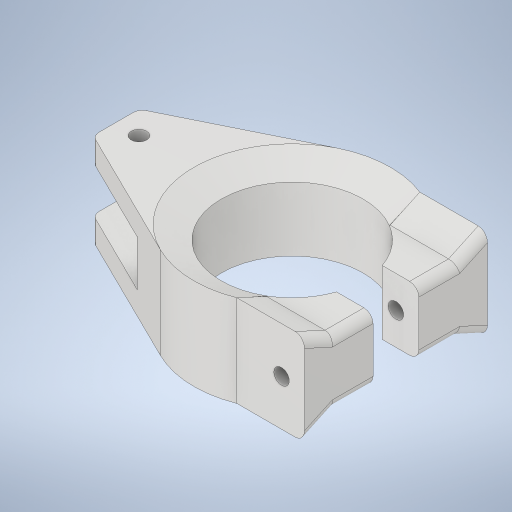
# Autodesk Inventor part: petbottlesfixingparts_sa
Saved by Autodesk Inventor 2024.1 (Build 281209000, 209)
## iProperties
Created: 2019-03-19
Part Number: petbottlesfixingparts_sa
Material: ABS プラスチック
Document SubType Name: Modeling
Designer: shun
Density: 1.06 g/cm^3
Appearance: 滑らか - 白
Author: shun
Autodesk Inventor part; units mm, degrees
ref_plane "YZ Plane" through (0, 0, 0) normal (1, 0, 0) x (0, 1, 0)
ref_plane "XZ Plane" through (0, 0, 0) normal (0, 1, 0) x (-1, 0, 0)
ref_plane "XY Plane" through (0, 0, 0) normal (0, 0, 1) x (1, 0, 0)
sketch "スケッチ1" plane through (0, 0, 0) normal (0, 1, 0) x (-1, 0, 0)
  circle A0 centre (0, 0) radius 15.5 construction
  circle A1 centre (0, 0) radius 21.5 construction
  line L0 (-22.6714, 5) -> (-14.6714, 5)
  line L1 (-14.6714, 5) -> (-14.6714, -5) construction
  line L2 (-14.6714, -5) -> (-22.6714, -5)
  line L3 (-22.6714, -5) -> (-22.6714, 5) construction
  line L4 (-22.6714, 5) -> (-14.6714, -5) construction
  line L5 (-14.6714, 5) -> (-22.6714, -5) construction
  line L6 (0, 0) -> (-18.6714, 0) construction
  line L7 (-22.6714, 5) -> (-22.6714, 20)
  line L8 (-22.6714, 20) -> (-7.8899, 20)
  line L9 (-22.6714, -5) -> (-22.6714, -20)
  line L10 (-22.6714, -20) -> (-7.8899, -20)
  arc A2 (-14.6714, -5) -> (-14.6714, 5) centre (0, 0) ccw
  line L11 (21.5, 0) -> (33.5, 0) construction
  line L12 (0, 0) -> (21.5, 0) construction
  line L13 (33.5, 0) -> (38.5, 0) construction
  line L14 (38.5, 0) -> (38.5, 5)
  line L15 (38.5, 0) -> (38.5, -5)
  line L16 (38.5, 5) -> (9.5018, 19.2864)
  line L17 (38.5, -5) -> (9.5018, -19.2864)
  arc A3 (9.5018, 19.2864) -> (-7.8899, 20) centre (0, 0) ccw
  arc A4 (-7.8899, -20) -> (9.5018, -19.2864) centre (0, 0) ccw
  dimension "d0" = 31
  dimension "d1" = 43
  dimension "d2" = 10
  dimension "d3" = 8
  dimension "d4" = 15
  dimension "d5" = 15
  dimension "d6" = 12
  dimension "d7" = 5
  dimension "d8" = 5
  dimension "d9" = 5
  constraints: 36 end point, 11 point on circle, 6 coincident, 5 horizontal, 4 centre point, 4 perpendicular, 2 midpoint, 2 parallel, 2 tangent, 2 vertical, 1 point on line, 3 other
  measures "d1" diameter of A1
  measures "d2" distance of L0.end L1.end
  measures "d3" distance of L1.end L2.end
  measures "d4" distance of L0.start L7.end
  measures "d5" distance of L2.end L9.end
  measures "d6" distance of L11.start L11.end
  measures "d7" distance of L13.start L13.end
  measures "d8" distance of L13.end L14.end
  measures "d9" distance of L13.end L15.end
extrude "押し出し1" add sketch "スケッチ1" along normal mid plane 20
sketch "スケッチ2" plane through (0, 0, 0) normal (0, 0, 1) x (1, 0, 0)
  line L0 (-38.5, -10) -> (-38.5, 10) projected
  line L1 (-19.5, -5) -> (-38.5, -5)
  line L2 (-38.5, -5) -> (-38.5, 5)
  line L3 (-38.5, 5) -> (-19.5, 5)
  line L4 (-19.5, 5) -> (-19.5, -5)
  line L5 (-19.5, -5) -> (-38.5, 5) construction
  line L6 (-38.5, -5) -> (-19.5, 5) construction
  line L7 (0, 0) -> (-29, 0) construction
  line L8 (-9.5018, -10) -> (-9.5018, 10) projected
  dimension "d12" = 10
  dimension "d13" = 19
  constraints: 14 end point, 2 midpoint, 2 parallel, 2 perpendicular, 1 horizontal, 1 point on line
  measures "d12" distance of L1.end L2.end
  measures "d13" distance of L2.end L3.end
extrude "押し出し2" cut sketch "スケッチ2" along normal mid plane 100
hole "穴1" at (-33.5, 0, 0) direction (0, -1, 0) diameter 3.4 end through all both
sketch "スケッチ3" plane through (7.8899, 10, 20) normal (0, 0, 1) x (1, 0, 0)
  line L0 (14.7815, 0) -> (6.7815, 0) projected
  line L1 (9.7815, 0) -> (9.7815, -20) construction
  line L2 (14.7815, -20) -> (0, -20) projected
  line L3 (14.7815, -20) -> (14.7815, 0) projected
  point P0 (-7.8899, -10)
  point P1 (9.7815, -10)
  dimension "d23" = 5
  constraints: 2 end point, 2 point on line, 1 midpoint, 1 vertical
  measures "d23" distance between parallel lines of L3 L1
hole "穴2" at (17.6714, 0, 20) direction (0, 0, -1) diameter 3.4 end through all both
chamfer "面取り1" distance 6 distance2 3 1 edges at (-15.5, 10, 0) measured on face at (-20.2308, 10, -11.0619)
sketch "スケッチ4" plane through (22.6714, -10, 5) normal (1, 0, 0) x (0, 0, -1)
  line L0 (-15, 0) -> (-15, 20) projected
  line L1 (0, 20) -> (-14.2864, 20) projected
  line L2 (-15, 20) -> (0, 20)
  line L3 (0, 20) -> (0, 0) projected
  line L4 (0, 20) -> (0, 17)
  line L5 (0, 17) -> (-8.5, 17)
  line L6 (0, 15) -> (-9.3606, 15) projected
  line L7 (-8.5, 17) -> (-15, 20)
  point P0 (5, 10)
  point P1 (-9.3606, 15)
  dimension "d34" = 3
  dimension "d35" = 8.5
  constraints: 8 end point, 1 collinear, 1 horizontal, 1 point on line, 1 other
  measures "d34" distance of L1.start L4.end
  measures "d35" distance of L4.end L5.end
extrude "押し出し3" cut sketch "スケッチ4" against normal blind 14.782
mirror "ミラー1" about plane through (0, 0, 0) normal (0, 0, 1) of "押し出し3"
chamfer "面取り2" distance 6 distance2 3 1 edges at (-15.5, -10, 0) measured on face at (-20.2308, -10, -11.0619)
mirror "ミラー2" about plane through (0, 0, 0) normal (0, 1, 0) of "押し出し3", "ミラー1"
fillet "フィレット1" radius 2 4 edges at (-38.5, -7.5, 5) (-38.5, 7.5, 5) (-38.5, 7.5, -5) (-38.5, -7.5, -5)
fillet "フィレット2" radius 2 8 edges at (22.6714, -7, 9.25) (22.6714, -8.5, 16.75) (22.6714, 7, 9.25) (22.6714, 8.5, 16.75) (22.6714, 8.5, -16.75) (22.6714, 7, -9.25) (22.6714, -7, -9.25) (22.6714, -8.5, -16.75)
equation "\"d9\" = d8"
